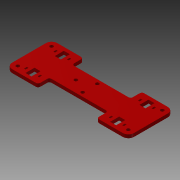
# Autodesk Inventor part: plastic_part_12
Saved by Autodesk Inventor 2013 (Build 170138000, 138)
## iProperties
Shininess: 20.0
Created: 2013-05-22
Part Number: plastic_part_12
Document SubType Name: Modeling
Designer: Noa Izumi
Material: Default
Density: 1 g/cm^3
Density: 0.0
Volumn: 0.0
Area: 0.0
PropertySet Name: Model Information
Control State: 0
Master: False
Checked Out: False
Author: Noa Izumi
Autodesk Inventor part; units mm, degrees
ref_plane "YZ Plane" through (0, 0, 0) normal (1, 0, 0) x (0, 1, 0)
ref_plane "XZ Plane" through (0, 0, 0) normal (0, 1, 0) x (-1, 0, 0)
ref_plane "XY Plane" through (0, 0, 0) normal (0, 0, 1) x (1, 0, 0)
sketch "Sketch1" plane through (0, 0, 0) normal (0, 0, 1) x (1, 0, 0)
  line L0 (0, 0) -> (108, 0)
  line L1 (108, 0) -> (108, 40)
  line L2 (108, 40) -> (0, 40)
  line L3 (0, 40) -> (0, 0)
  line L4 (13.854, 37) -> (19.146, 37)
  line L5 (19.146, 37) -> (19.146, 29)
  line L6 (19.146, 29) -> (13.854, 29)
  line L7 (13.854, 29) -> (13.854, 37)
  line L8 (13.854, 11) -> (19.146, 11)
  line L9 (19.146, 11) -> (19.146, 3)
  line L10 (19.146, 3) -> (13.854, 3)
  line L11 (13.854, 3) -> (13.854, 11)
  line L12 (88.854, 37) -> (94.146, 37)
  line L13 (94.146, 37) -> (94.146, 29)
  line L14 (94.146, 29) -> (88.854, 29)
  line L15 (88.854, 29) -> (88.854, 37)
  line L16 (88.854, 11) -> (94.146, 11)
  line L17 (94.146, 11) -> (94.146, 3)
  line L18 (94.146, 3) -> (88.854, 3)
  line L19 (88.854, 3) -> (88.854, 11)
  dimension "d0" = 40
  dimension "d1" = 108
  dimension "d73" = 8
  dimension "d74" = 5.292
  dimension "d75" = 3
  dimension "d76" = 13.854
  dimension "d77" = 5.292
  dimension "d78" = 8
  dimension "d79" = 3
  dimension "d80" = 5.292
  dimension "d81" = 8
  dimension "d82" = 13.854
  dimension "d83" = 3
  dimension "d84" = 5.292
  dimension "d85" = 13.854
  constraints: 40 end point, 10 parallel, 5 horizontal, 5 perpendicular, 2 point on line
  measures "d0" distance of L2.end L0.start
  measures "d1" distance of L0.start L0.end
  measures "d73" distance of L6.end L4.start
  measures "d74" distance of L4.start L4.end
  measures "d75" distance between parallel lines of L4 L2
  measures "d76" distance between parallel lines of L3 L7
  measures "d77" distance of L9.end L10.end
  measures "d78" distance of L10.end L8.start
  measures "d79" distance between parallel lines of L0 L10
  measures "d80" distance of L12.start L12.end
  measures "d81" distance of L14.end L12.start
  measures "d82" distance between parallel lines of L1 L13
  measures "d83" distance between parallel lines of L12 L2
  measures "d84" distance of L17.end L18.end
  measures "d85" distance between parallel lines of L1 L17
extrude "Extrusion1" add sketch "Sketch1" along normal blind 3
sketch "Sketch3" plane through (0, 0, 3) normal (0, 0, 1) x (1, 0, 0)
  line L0 (0, 0) -> (0, 40) projected
  line L1 (108, 0) -> (0, 0) projected
  line L2 (0, 40) -> (108, 40) projected
  point P0 (54, 26.5)
  point P1 (54, 13.5)
  dimension "d56" = 54
  dimension "d57" = 13.5
  dimension "d58" = 13.5
  dimension "d59" = 54
  measures "d56" distance from line of point (54, 26.5) L0
  measures "d57" distance from line of L2 point (54, 26.5)
  measures "d58" distance from line of L1 point (54, 13.5)
  measures "d59" distance from line of point (54, 13.5) L0
hole "Hole1" at (54, 26.5, 3) at (54, 13.5, 3) direction (0, 0, -1) diameter 3 end through all
sketch "Sketch8" plane through (0, 0, 3) normal (0, 0, 1) x (1, 0, 0)
  line L0 (108, 0) -> (0, 0) projected
  line L1 (0, 40) -> (108, 40) projected
  line L2 (28, 40) -> (80, 40)
  line L3 (80, 40) -> (80, 30)
  line L4 (80, 30) -> (28, 30)
  line L5 (28, 30) -> (28, 40)
  line L6 (28, 0) -> (80, 0)
  line L7 (80, 0) -> (80, 10)
  line L8 (80, 10) -> (28, 10)
  line L9 (28, 10) -> (28, 0)
  line L10 (108, 40) -> (108, 0) projected
  line L11 (0, 0) -> (0, 40) projected
  dimension "d68" = 10
  dimension "d69" = 10
  dimension "d87" = 28
  dimension "d88" = 28
  dimension "d130" = 28
  dimension "d131" = 28
  constraints: 16 end point, 4 parallel, 2 horizontal, 2 perpendicular, 2 point on line
  measures "d68" distance between parallel lines of L2 L4
  measures "d69" distance of L8.end L6.start
  measures "d87" distance between parallel lines of L10 L3
  measures "d88" distance between parallel lines of L10 L7
  measures "d130" distance between parallel lines of L5 L11
  measures "d131" distance between parallel lines of L9 L11
extrude "Extrusion5" cut sketch "Sketch8" against normal through all contours L0 L9 L8 L7 | L3 L4 L5 L1
fillet "Fillet3" radius 2 8 edges at (28, 40, 1.5) (28, 0, 1.5) (28, 10, 1.5) (28, 30, 1.5) (80, 10, 1.5) (80, 30, 1.5) (80, 0, 1.5) (80, 40, 1.5)
fillet "Fillet4" radius 5 4 edges at (0, 0, 1.5) (0, 40, 1.5) (108, 0, 1.5) (108, 40, 1.5)
sketch "Sketch12" plane through (0, 0, 3) normal (0, 0, 1) x (1, 0, 0)
  arc A0 (5, 40) -> (0, 35) centre (5, 35) ccw projected
  arc A1 (0, 5) -> (5, 0) centre (5, 5) ccw projected
  arc A2 (103, 0) -> (108, 5) centre (103, 5) ccw projected
  arc A3 (108, 35) -> (103, 40) centre (103, 35) ccw projected
  circle A4 centre (54, 26.5) radius 1.5 projected
  line L0 (78, 30) -> (30, 30) projected
  point P0 (41.5, 20)
  dimension "d141" = 12.5
  dimension "d142" = 10
  constraints: 4 coincident
  measures "d141" horizontal distance of A4.centre point (41.5, 20)
  measures "d142" distance from line of point (41.5, 20) L0
hole "Hole4" at (5, 35, 3) at (5, 5, 3) at (103, 35, 3) at (103, 5, 3) at (41.5, 20, 3) direction (0, 0, -1) diameter 3 end through all
sketch "草圖14" plane through (0, 0, 3) normal (0, 0, 1) x (1, 0, 0)
  line L0 (94.146, 37) -> (94.146, 29) projected
  line L1 (88.854, 29) -> (88.854, 37) projected
  line L2 (19.146, 37) -> (19.146, 29) projected
  line L3 (13.854, 29) -> (13.854, 37) projected
  line L4 (13.854, 37) -> (19.146, 37) projected
  line L5 (13.854, 11) -> (19.146, 11) projected
  line L6 (9.8, 34.25) -> (11.2, 34.25)
  line L7 (11.2, 34.25) -> (11.2, 31.75)
  line L8 (11.2, 31.75) -> (9.8, 31.75)
  line L9 (9.8, 31.75) -> (9.8, 34.25)
  line L10 (21.8, 34.25) -> (23.2, 34.25)
  line L11 (23.2, 34.25) -> (23.2, 31.75)
  line L12 (23.2, 31.75) -> (21.8, 31.75)
  line L13 (21.8, 31.75) -> (21.8, 34.25)
  line L14 (9.8, 8.25) -> (11.2, 8.25)
  line L15 (11.2, 8.25) -> (11.2, 5.75)
  line L16 (11.2, 5.75) -> (9.8, 5.75)
  line L17 (9.8, 5.75) -> (9.8, 8.25)
  line L18 (21.8, 8.25) -> (23.2, 8.25)
  line L19 (23.2, 8.25) -> (23.2, 5.75)
  line L20 (23.2, 5.75) -> (21.8, 5.75)
  line L21 (21.8, 5.75) -> (21.8, 8.25)
  line L22 (84.8, 34.25) -> (86.2, 34.25)
  line L23 (86.2, 34.25) -> (86.2, 31.75)
  line L24 (86.2, 31.75) -> (84.8, 31.75)
  line L25 (84.8, 31.75) -> (84.8, 34.25)
  line L26 (96.8, 34.25) -> (98.2, 34.25)
  line L27 (98.2, 34.25) -> (98.2, 31.75)
  line L28 (98.2, 31.75) -> (96.8, 31.75)
  line L29 (96.8, 31.75) -> (96.8, 34.25)
  line L30 (84.8, 8.25) -> (86.2, 8.25)
  line L31 (86.2, 8.25) -> (86.2, 5.75)
  line L32 (86.2, 5.75) -> (84.8, 5.75)
  line L33 (84.8, 5.75) -> (84.8, 8.25)
  line L34 (96.8, 8.25) -> (98.2, 8.25)
  line L35 (98.2, 8.25) -> (98.2, 5.75)
  line L36 (98.2, 5.75) -> (96.8, 5.75)
  line L37 (96.8, 5.75) -> (96.8, 8.25)
  point P0 (0, 0)
  dimension "d143" = 1.4
  dimension "d145" = 2.654
  dimension "d146" = 2.75
  dimension "d147" = 2.5
  dimension "d148" = 1.4
  dimension "d149" = 2.654
  dimension "d150" = 2.5
  dimension "d151" = 1.4
  dimension "d152" = 2.75
  dimension "d153" = 1.4
  dimension "d154" = 2.5
  dimension "d155" = 2.654
  dimension "d156" = 2.654
  dimension "d157" = 1.4
  dimension "d158" = 1.4
  dimension "d159" = 1.4
  constraints: 64 end point, 16 parallel, 8 horizontal, 8 perpendicular, 2 point on line
  measures "d143" distance of L6.start L6.end
  measures "d145" distance between parallel lines of L3 L7
  measures "d146" distance between parallel lines of L4 L6
  measures "d147" distance of L8.end L6.start
  measures "d148" distance of L10.start L10.end
  measures "d149" distance between parallel lines of L13 L2
  measures "d150" distance of L16.end L14.start
  measures "d151" distance of L14.start L14.end
  measures "d152" distance between parallel lines of L5 L14
  measures "d153" distance of L22.start L22.end
  measures "d154" distance of L24.end L22.start
  measures "d155" distance between parallel lines of L1 L23
  measures "d156" distance between parallel lines of L0 L29
  measures "d157" distance of L26.start L26.end
  measures "d158" distance of L31.end L32.end
  measures "d159" distance of L35.end L36.end
extrude "擠出7" cut sketch "草圖14" against normal through all
